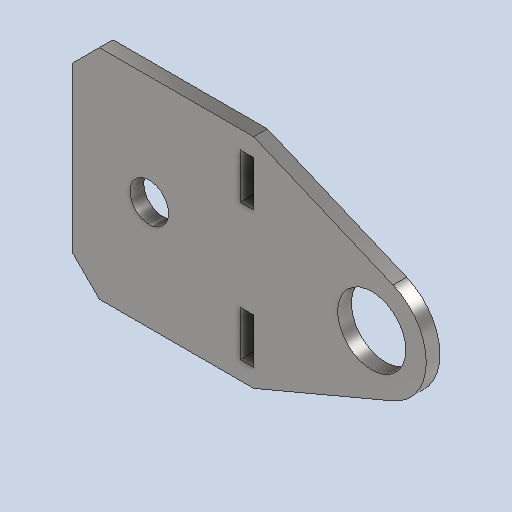
# Autodesk Inventor part: A_beam_piston_mount_2
Saved by Autodesk Inventor 2025.2 (Build 292293000, 293)
## iProperties
Created: 2025-05-02
Part Number: A_beam_piston_mount_2
Material: Stainless Steel
Document SubType Name: Sheet Metal
Designer: Caspe
Density: 8 g/cm^3
Sheet Metal Rule: Default_mm
Appearance: Semi-Polished
Flat Pattern Width: 7.8 cm
Flat Pattern Length: 4.8 cm
Flat Pattern Area: 37.44 cm^2
Sheet Metal Width: 78,000 mm
Sheet Metal Length: 48,000 mm
Sheet Metal Area: 3744,000 mm^2
Mass: 66.7838 g
Surface Area: 65.8977 cm^2
Volume: 8.34798 cm^3
Author: Caspe
Autodesk Inventor part; units mm, degrees
ref_plane "YZ Plane" through (0, 0, 0) normal (1, 0, 0) x (0, 1, 0)
ref_plane "XZ Plane" through (0, 0, 0) normal (0, 1, 0) x (-1, 0, 0)
ref_plane "XY Plane" through (0, 0, 0) normal (0, 0, 1) x (1, 0, 0)
sketch "Sketch1" plane through (0, 0, 0) normal (0, 0, 1) x (1, 0, 0)
  line L0 (0, 0) -> (40, 0)
  line L1 (40, 0) -> (40, 40)
  line L2 (40, 40) -> (0, 40)
  line L3 (0, 40) -> (0, 0)
  line L4 (40, 0) -> (37, 0)
  line L5 (37, 0) -> (37, 10)
  line L6 (37, 10) -> (40, 10)
  line L7 (40, 10) -> (40, 0)
  line L8 (40, 40) -> (37, 40)
  line L9 (37, 40) -> (37, 30)
  line L10 (37, 30) -> (40, 30)
  line L11 (40, 30) -> (40, 40)
  line L12 (0, -4) -> (40, -4)
  line L13 (40, -4) -> (40, 44)
  line L14 (40, 44) -> (0, 44)
  line L15 (0, 44) -> (0, -4)
  circle A0 centre (66, 20) radius 7.5
  circle A1 centre (66, 20) radius 12
  line L16 (40, -4) -> (70.6666, 8.9445)
  line L17 (40, 20) -> (43.7791, 20)
  line L18 (40, 44) -> (70.6666, 31.0555)
  circle A2 centre (17, 20) radius 4.25
  line L19 (37, 30) -> (37, 10)
  point P0 (20, 40)
  dimension "d0" = 40
  dimension "d1" = 40
  dimension "d2" = 3
  dimension "d3" = 10
  dimension "d4" = 10
  dimension "d5" = 4
  dimension "d6" = 4
  dimension "d7" = 15
  dimension "d8" = 24
  dimension "d9" = 26
  dimension "d11" = 8.5
  dimension "d17" = 20
  dimension "d18" = 20
  measures "d0" distance of L2.end L1.end
  measures "d1" distance of L1.end L0.end
  measures "d2" distance of L5.end L6.end
  measures "d3" distance of L4.end L5.end
  measures "d4" distance of L9.end L8.end
  measures "d5" distance between parallel lines of L14 L2
  measures "d6" distance between parallel lines of L0 L12
  measures "d7" diameter of A0
  measures "d8" diameter of A1
  measures "d9" distance from line of A1.centre L1
  measures "d11" diameter of A2
  measures "d17" distance from line of L19 A2.centre
  measures "d18" distance from line of L2 A2.centre
extrude "Plate1" add sketch "Sketch1" along normal blind 3 contours L3 L2 L9 L19 L5 L0 | L0 L13 L12 L15 | L15 L14 L13 L2 | L1 L13 L18 A1 L16 | L19 L10 L1 L6 | A1
chamfer "Corner Chamfer1" distance 6 angle 45 2 edges at (0, 44, 1.5) (0, -4, 1.5)
equation "\"d6\" = d5"
equation "\"d10\" = Thickness"
equation "\"BendRadius\" = Thickness"
equation "\"BendReliefWidth\" = Thickness"
equation "\"BendReliefDepth\" = 0.5 * Thickness"
equation "\"CornerReliefSize\" = 4 * Thickness"
equation "\"MinimumRemnant\" = 2 * Thickness"
equation "\"TransitionRadius\" = BendRadius"
equation "\"JacobiRadiusSize\" = BendRadius"
equation "\"GapSize\" = Thickness"
equation "\"Thickness\" = 3"
body "Solid1"
